cale (Autodesk Fusion 360 design; units mm, degrees)
Autodesk Fusion 360 part; units mm, degrees
sketch "Sketch1" plane through (0, 0, 0) normal (0, 0, 1) x (1, 0, 0)
  line L0 (11.5, 4) -> (-11.5, 4)
  line L1 (-11.5, 4) -> (-11.5, -4)
  line L2 (-11.5, -4) -> (11.5, -4)
  line L3 (11.5, -4) -> (11.5, 4)
  line L4 (11.5, 4) -> (-11.5, -4) construction
  line L5 (-11.5, 4) -> (11.5, -4) construction
  line L6 (-11.5, 4) -> (11.5, 4)
  line L7 (11.5, 4) -> (11.5, 2.4)
  line L8 (11.5, 2.4) -> (-11.5, 2.4)
  line L9 (-11.5, 2.4) -> (-11.5, 4)
  dimension "d1" = 23
  dimension "d2" = 8
  dimension "d3" = 1.6
  measures "d1" distance of L1.end L2.end
  measures "d2" distance of L0.end L1.end
  measures "d3" distance of L0.end L8.end
extrude "Extrude1" add sketch "Sketch1" along normal blind 1.6
extrude "Extrude2" add sketch "Sketch1" along normal blind 15 contours L0 L1 L3 L6 L7 L8 L9
hole "Hole1" at (-6.5, 2.4, 10) direction (0, 1, 0) diameter 3.4 depth 9 tip angle 118
hole "Hole2" at (6.5, 2.4, 10) direction (0, 1, 0) diameter 3.4 depth 12 tip angle 118
sketch "Sketch2" plane through (0, 0, 0) normal (1, 0, 0) x (0, 1, 0)
  line L0 (2.4, 1.6) -> (-4, 1.6)
  line L1 (-4, 1.6) -> (2.4, 1.6)
  line L2 (2.4, 1.6) -> (2.4, 15)
  line L3 (-3.1915, 1.6) -> (2.4, 7.2966)
  line L4 (2.4, 1.6) -> (-3.1915, 1.6)
extrude "Extrude3" add sketch "Sketch2" along normal blind 1.6 from surface at -9.6
extrude "Extrude4" add sketch "Sketch2" along normal blind 1.6 from surface at -0.8
extrude "Extrude5" add sketch "Sketch2" along normal blind 1.6 from surface at 8
named bodies: "Clapet"
